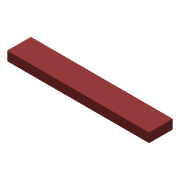
# Autodesk Inventor part: PROGRAM
Saved by Autodesk Inventor 2017 (Build 210142000, 142)
## iProperties
Part Number: PROGRAM
Material: Generisch
Document SubType Name: Modeling
Designer: Werkstatt
Density: 1 g/cm^3
Appearance: 1X06-SMD, PROGRAM
Author: Werkstatt
Autodesk Inventor part; units mm, degrees
ref_plane "YZ Plane" through (0, 0, 0) normal (1, 0, 0) x (0, 1, 0)
ref_plane "XZ Plane" through (0, 0, 0) normal (0, 1, 0) x (-1, 0, 0)
ref_plane "XY Plane" through (0, 0, 0) normal (0, 0, 1) x (1, 0, 0)
sketch "1X06-SMD, PROGRAM_35" plane through (0, 0, 0) normal (0, 0, 1) x (1, 0, 0)
  line L0 (-7.6835, 1.3135) -> (7.6835, 1.3135)
  line L1 (7.6835, 1.3135) -> (7.6835, -1.25)
  line L2 (7.6835, -1.25) -> (-7.6835, -1.25)
  line L3 (-7.6835, -1.25) -> (-7.6835, 1.3135)
  constraints: 8 end point
extrude "Extrusion1" add sketch "1X06-SMD, PROGRAM_35" along normal blind 1
